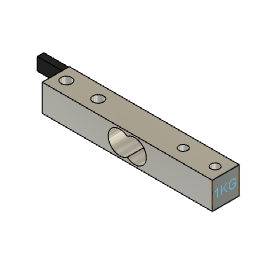
Testbench_BLDC_complete (Autodesk Fusion 360 archive; units mm, degrees)
design "LoadCell_1kg"
Autodesk Fusion 360 part; units mm, degrees
sketch "Skizze1" plane through (0, 0, 0) normal (0, 0, 1) x (1, 0, 0)
  line L0 (0, 0) -> (80, 0)
  line L1 (80, 0) -> (80, 12.7)
  line L2 (80, 12.7) -> (0, 12.7)
  line L3 (0, 12.7) -> (0, 0)
  line L4 (40, 12.7) -> (40, 0) construction
  circle A0 centre (20, 6.35) radius 2.5
  circle A1 centre (5, 6.35) radius 2.5
  circle A2 centre (60, 6.35) radius 2
  circle A3 centre (75, 6.35) radius 2
  line L5 (0, 6.35) -> (80, 6.35) construction
  dimension "d1" = 80
  dimension "d2" = 12.7
  dimension "d3" = 20
  dimension "d4" = 15
  dimension "d5" = 15
  dimension "d6" = 20
  dimension "d7" = 4
  dimension "d8" = 4
  dimension "d9" = 5
  dimension "d10" = 5
  constraint horizontal L0
  constraint vertical L1
  constraint horizontal L2
  constraint vertical L3
  constraint coincident L0.start L3.end
  constraint midpoint L2 L4.start
  constraint midpoint L0 L4.end
  constraint midpoint L3 L5.start
  constraint midpoint L1 L5.end
  constraint coincident A3.centre L5
  constraint coincident A2.centre L5
  constraint coincident A0.centre L5
  constraint coincident A1.centre L5
  measures "d1" distance of L0.start L0.end
  measures "d2" distance of L0.start L2.end
  measures "d3" distance of L4 A0.centre
  measures "d4" horizontal distance of A0.centre A1.centre
  measures "d5" distance of A2.centre A3.centre
  measures "d6" distance of L4 A2.centre
  measures "d7" diameter of A2
  measures "d8" diameter of A3
  measures "d9" diameter of A0
  measures "d10" diameter of A1
extrude "Extrusion1" add sketch "Skizze1" along normal blind 12.7
sketch "Skizze2" plane through (0, 0, 0) normal (0, -1, 0) x (1, 0, 0)
  line L0 (0, 0) -> (80, 0)
  line L1 (80, 0) -> (80, 12.7)
  line L2 (80, 12.7) -> (0, 12.7)
  line L3 (0, 12.7) -> (0, 0)
  line L4 (40, 12.7) -> (40, 0) construction
  circle A0 centre (36.5, 6.35) radius 5.5
  circle A1 centre (43.5, 6.35) radius 5.5
  line L5 (0, 6.35) -> (80, 6.35)
  line L6 (36.5, 6.35) -> (43.5, 6.35)
  point P0 (40, 6.35)
  point P1 (40, 6.35)
  dimension "d13" = 11
  dimension "d14" = 11
  dimension "d15" = 7
  constraint midpoint L2 L4.start
  constraint midpoint L0 L4.end
  constraint midpoint L3 L5.start
  constraint midpoint L1 L5.end
  constraint coincident A1.centre L5
  constraint coincident A0.centre L5
  constraint coincident A0.centre L6.start
  constraint coincident A1.centre L6.end
  constraint midpoint L6 P1
  constraint midpoint L5 P1
  constraint coincident P1 P0
  measures "d13" diameter of A1
  measures "d14" diameter of A0
  measures "d15" distance of A0.centre A1.centre
extrude "Extrusion2" cut sketch "Skizze2" against normal through all contours A0 A1 L5 L6 | A0 A1 L5 L6 | A0 A1 L5 L6 | A0 A1 L5 L6 | A0 A1 L5 L6 | A0 A1 L5 L6
sketch "Skizze3" plane through (0, 12.7, 0) normal (0, 1, 0) x (-1, 0, 0)
  arc A0 (-40, 10.5926) -> (-40, 2.1074) centre (-43.5, 6.35) ccw
  arc A1 (-40, 2.1074) -> (-40, 10.5926) centre (-36.5, 6.35) ccw
  line L0 (-80, 0) -> (0, 0)
  line L1 (0, 0) -> (0, 12.7)
  line L2 (0, 12.7) -> (-80, 12.7)
  line L3 (-80, 12.7) -> (-80, 0)
  line L4 (-25, 9.35) -> (15, 9.35)
  line L5 (15, 9.35) -> (15, 3.35)
  line L6 (15, 3.35) -> (-25, 3.35)
  line L7 (-25, 3.35) -> (-25, 9.35)
  point P0 (-25, 6.35)
  point P1 (0, 6.35)
  dimension "d17" = 6
  dimension "d18" = 40
  dimension "d19" = 15
  constraint horizontal L4
  constraint vertical L5
  constraint horizontal L6
  constraint vertical L7
  constraint midpoint L7 P0
  constraint midpoint L1 P1
  constraint horizontal P0 P1
  measures "d17" distance of L4.start L6.end
  measures "d18" distance of L4.start L4.end
  measures "d19" distance of L1 L5
extrude "Extrusion3" add sketch "Skizze3" along normal blind 3 contours L1 L4 L6 L7 | L1 L4 L5 L6
sketch "Skizze4" plane through (80, 0, 0) normal (1, 0, 0) x (0, 1, 0)
  line L0 (0, 0) -> (12.7, 0)
  line L1 (12.7, 0) -> (12.7, 12.7)
  line L2 (12.7, 12.7) -> (0, 12.7)
  line L3 (0, 12.7) -> (0, 0)
  line L4 (0, 0) -> (12.7, 0) construction
  line L5 (12.7, 0) -> (12.7, 12.7) construction
  line L6 (12.7, 12.7) -> (0, 12.7) construction
  line L7 (0, 12.7) -> (0, 0) construction
  dimension "d22" = 4
  constraint midpoint L2
  constraint midpoint L0
equation "d15 = 18 mm - 11 mm"

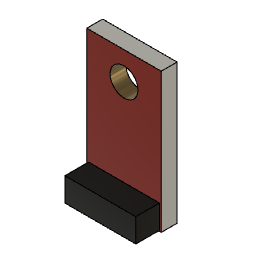
design "SparkFun Analog Line Sensor Breakout - QRE1113"
Autodesk Fusion 360 part; units mm, degrees
sketch "Skizze1" plane through (0, 0, 0) normal (0, 1, 0) x (1, 0, 0)
  line L0 (0, 0) -> (8, 0)
  line L1 (8, 0) -> (8, -15)
  line L2 (8, -15) -> (0, -15)
  line L3 (0, -15) -> (0, 0)
  circle A0 centre (4, -12) radius 1.5
  line L4 (2.6, -9) -> (5.4, -9)
  line L5 (5.4, -9) -> (5.4, -5.8)
  line L6 (5.4, -5.8) -> (2.6, -5.8)
  line L7 (2.6, -5.8) -> (2.6, -9)
  line L8 (0.19, -2.64) -> (7.81, -2.64)
  line L9 (7.81, -2.64) -> (7.81, -0.1)
  line L10 (7.81, -0.1) -> (0.19, -0.1)
  line L11 (0.19, -0.1) -> (0.19, -2.64)
  point P0 (4, -15)
  point P1 (4, -9)
  point P2 (4, -2.64)
  dimension "d1" = 8
  dimension "d2" = 15
  dimension "d3" = 3
  dimension "d4" = 3
  dimension "d5" = 2.8
  dimension "d6" = 3.2
  dimension "d7" = 6
  dimension "d8" = 7.62
  dimension "d9" = 2.54
  dimension "d10" = 0.1
  constraint horizontal L0
  constraint vertical L1
  constraint horizontal L2
  constraint vertical L3
  constraint coincident L0.start L3.end
  constraint midpoint L2 P0
  constraint vertical A0.centre P0
  constraint horizontal L4
  constraint vertical L5
  constraint horizontal L6
  constraint vertical L7
  constraint midpoint L4 P1
  constraint vertical P0 P1
  constraint horizontal L8
  constraint vertical L9
  constraint horizontal L10
  constraint vertical L11
  constraint midpoint L8 P2
  constraint vertical P0 P2
  measures "d1" distance of L0.start L0.end
  measures "d2" distance of L0.start L2.end
  measures "d3" diameter of A0
  measures "d4" distance of L2 A0.centre
  measures "d5" distance of L4.start L4.end
  measures "d6" distance of L4.start L6.end
  measures "d7" distance of L2 L4
  measures "d8" distance of L8.start L8.end
  measures "d9" distance of L8.start L10.end
  measures "d10" distance of L0 L10
extrude "Extrusion1" add sketch "Skizze1" against normal blind 1.7 contours L0 L1 L2 L3 | L4 L5 L6 L7 | L8 L9 L10 L11
extrude "Extrusion2" add sketch "Skizze1" along normal blind 1.7 contours L4 L5 L6 L7
extrude "Extrusion3" add sketch "Skizze1" against normal blind 4.24 contours L8 L9 L10 L11
equation "d4 = 1.5 mm + 1.5 mm"
equation "d8 = 2.54 * 3 mm"
equation "d15 = -1.7 mm - 2.54 mm"

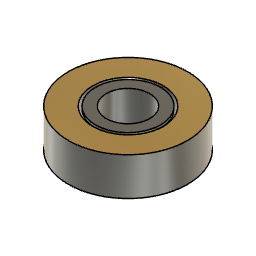
design "Kugellager_608-2Z"
Autodesk Fusion 360 part; units mm, degrees
sketch "Skizze1" plane through (0, 0, 0) normal (0, 0, 1) x (1, 0, 0)
  circle A0 centre (0, 0) radius 4
  circle A1 centre (0, 0) radius 11
  circle A2 centre (0, 0) radius 6
  dimension "d1" = 8
  dimension "d2" = 22
  dimension "d9" = 12
  constraint coincident A0.centre A1.centre
  measures "d1" diameter of A0
  measures "d2" diameter of A1
  measures "d9" diameter of A2
extrude "Extrusion1" add sketch "Skizze1" along normal blind 7 contours A1 makes body 1
extrude "Extrusion2" add sketch "Skizze1" along normal blind 7 separate body contours A2 makes body 2
chamfer "Fase3" distance 0.5 distance2 0.5 2 edges at (-5.594, 2.1697, 7) (-5.594, 2.1697, 0) measured on face at (9.2924, -0.5465, 7) measured on face at (5.9702, -0.5974, 4.6667) on bodies 1

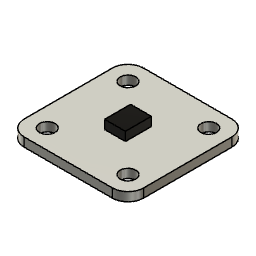
design "AS5600"
Autodesk Fusion 360 part; units mm, degrees
sketch "Skizze1" plane through (0, 0, 0) normal (0, 0, 1) x (1, 0, 0)
  line L0 (11.5, -11.5) -> (-11.5, -11.5)
  line L1 (-11.5, -11.5) -> (-11.5, 11.5)
  line L2 (-11.5, 11.5) -> (11.5, 11.5)
  line L3 (11.5, 11.5) -> (11.5, -11.5)
  line L4 (11.5, -11.5) -> (-11.5, 11.5) construction
  line L5 (-11.5, -11.5) -> (11.5, 11.5) construction
  line L6 (2, -2.5) -> (-2, -2.5)
  line L7 (-2, -2.5) -> (-2, 2.5)
  line L8 (-2, 2.5) -> (2, 2.5)
  line L9 (2, 2.5) -> (2, -2.5)
  line L10 (2, -2.5) -> (-2, 2.5) construction
  line L11 (-2, -2.5) -> (2, 2.5) construction
  circle A0 centre (-7.7782, -7.7782) radius 1.5
  circle A1 centre (7.7782, -7.7782) radius 1.5
  circle A2 centre (7.7782, 7.7782) radius 1.5
  circle A3 centre (-7.7782, 7.7782) radius 1.5
  dimension "d1" = 23
  dimension "d2" = 23
  dimension "d3" = 4
  dimension "d4" = 5
  dimension "d5" = 3
  dimension "d6" = 11
  dimension "d8" = 360
  constraint horizontal L0
  constraint perpendicular L0 L1
  constraint parallel L0 L2
  constraint parallel L1 L3
  constraint coincident L4 origin
  constraint coincident L5 origin
  constraint horizontal L6
  constraint perpendicular L6 L7
  constraint parallel L6 L8
  constraint parallel L7 L9
  constraint coincident L10 origin
  constraint coincident L11 origin
  constraint coincident L5 A0.centre
  measures "d1" distance of L1.end L2.end
  measures "d2" distance of L0.end L1.end
  measures "d3" distance of L7.end L8.end
  measures "d4" distance of L6.end L7.end
  measures "d5" diameter of A0
  measures "d6" distance of origin A0.centre
extrude "Extrusion1" add sketch "Skizze1" against normal blind 1.7 contours L0 L1 L2 L3 | L6 L7 L8 L9
extrude "Extrusion2" add sketch "Skizze1" along normal blind 1.7 contours L6 L7 L8 L9
fillet "Abrundung1" radius 3 4 edges at (11.5, -11.5, -0.85) (-11.5, -11.5, -0.85) (-11.5, 11.5, -0.85) (11.5, 11.5, -0.85)
equation "d6 = ( ( 19 / 2 ) * 1 mm ) + 1.5 mm"
